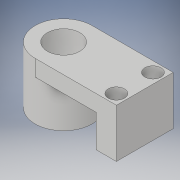
# Autodesk Inventor part: bedtiedown
Saved by Autodesk Inventor 2019.1 (Build 231200000, 200)
## iProperties
Created: 2019-08-29
Part Number: bedtiedown
Material: Generic
Document SubType Name: Modeling
Designer: Computus
Density: 1 g/cm^3
Appearance: Default
Author: Computus
Autodesk Inventor part; units mm, degrees
ref_plane "YZ Plane" through (0, 0, 0) normal (1, 0, 0) x (0, 1, 0)
ref_plane "XZ Plane" through (0, 0, 0) normal (0, 1, 0) x (-1, 0, 0)
ref_plane "XY Plane" through (0, 0, 0) normal (0, 0, 1) x (1, 0, 0)
sketch "Sketch1" plane through (0, 0, 0) normal (0, 1, 0) x (-1, 0, 0)
  circle A0 centre (0, 0) radius 4
  circle A1 centre (0, 0) radius 7
  dimension "d0" = 8
  dimension "d1" = 14
  constraints: 2 centre point, 2 coincident
  measures "d0" diameter of A0
  measures "d1" diameter of A1
extrude "Extrusion1" add sketch "Sketch1" along normal blind 10
sketch "Sketch2" plane through (0, 10, 0) normal (0, 1, 0) x (1, 0, 0)
  circle A0 centre (0, 0) radius 7 projected
  line L0 (0, -7) -> (20, -7)
  line L1 (0, 7) -> (20, 7)
  line L2 (20, 7) -> (20, -7)
  circle A1 centre (0, 0) radius 4
  arc A2 (0, 7) -> (0, -7) centre (0, 0) ccw
  dimension "d4" = 20
  constraints: 6 end point, 4 point on circle, 2 centre point, 2 coincident, 2 horizontal, 2 tangent, 1 perpendicular
  measures "d4" distance of L0.start L0.end
extrude "Extrusion2" add sketch "Sketch2" along normal blind 4
sketch "Sketch3" plane through (0, 10, 0) normal (0, -1, 0) x (1, 0, 0)
  line L0 (20, 7) -> (20, -7) projected
  line L1 (0, 7) -> (20, 7) projected
  line L2 (20, -7) -> (15, -7)
  line L3 (15, -7) -> (15, 7)
  line L4 (15, 7) -> (20, 7)
  line L5 (20, 7) -> (20, -7)
  point P0 (0, 0)
  dimension "d9" = 5
  constraints: 8 end point, 2 parallel, 1 horizontal, 1 perpendicular, 1 point on line
  measures "d9" distance of L3.end L4.end
extrude "Extrusion3" add sketch "Sketch3" along normal blind 8
sketch "Sketch4" plane through (0, 2, 0) normal (0, -1, 0) x (1, 0, 0)
  circle A0 centre (17.5, -4.5) radius 2
  line L0 (20, -7) -> (20, 7) projected
  circle A1 centre (17.5, 4.5) radius 2
  line L1 (20, 7) -> (15, 7) projected
  line L2 (15, -7) -> (20, -7) projected
  point P0 (0, 0)
  dimension "d12" = 4
  dimension "d13" = 2.5
  dimension "d14" = 4
  dimension "d15" = 2.5
  dimension "d16" = 2.5
  constraints: 2 centre point
  measures "d12" diameter of A0
  measures "d13" distance from line of L0 A0.centre
  measures "d14" diameter of A1
  measures "d15" distance from line of L1 A1.centre
  measures "d16" distance from line of L2 A0.centre
extrude "Extrusion4" cut sketch "Sketch4" against normal blind 15
body "Solid1"
